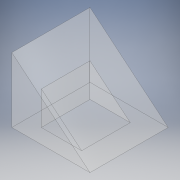
# Autodesk Inventor part: Transparent Grey Peice
Saved by Autodesk Inventor 2017 (Build 210142000, 142)
## iProperties
Created: 2018-05-17
Part Number: Transparent Grey Peice
Material: ABS Plastic
Document SubType Name: Modeling
Designer: 19000369
Density: 1.06 g/cm^3
Appearance: Clear
Author: 19000369
Autodesk Inventor part; units mm, degrees
ref_plane "YZ Plane" through (0, 0, 0) normal (1, 0, 0) x (0, 1, 0)
ref_plane "XZ Plane" through (0, 0, 0) normal (0, 1, 0) x (-1, 0, 0)
ref_plane "XY Plane" through (0, 0, 0) normal (0, 0, 1) x (1, 0, 0)
sketch "Sketch1" plane through (0, 0, 0) normal (0, 0, 1) x (1, 0, 0)
  line L0 (0, 0) -> (0, 6.4719)
  line L1 (0, 0) -> (7.7978, 0)
  line L2 (7.7978, 0) -> (0, 6.4719)
  dimension "d0" = 6.4719
  dimension "d1" = 7.7978
  constraints: 6 end point, 1 horizontal, 1 vertical
  measures "d0" distance of L0.start L0.end
  measures "d1" distance of L0.start L1.end
extrude "Extrusion1" add sketch "Sketch1" along normal blind 7.7978
shell "Shell1" thickness 1.4732 removed faces 1 at (5.1985, 0, 2.5993)
body "Solid1"
